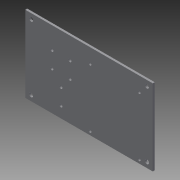
# Autodesk Inventor part: base_ps_rpi
Saved by Autodesk Inventor 2014 (Build 180170000, 170)
## iProperties
Created: 2015-04-20
Part Number: base_ps_rpi
Material: Generic
Document SubType Name: Modeling
Designer: Sousaadm
Density: 1 g/cm^3
Appearance: Default
Author: Sousaadm
Autodesk Inventor part; units mm, degrees
ref_plane "YZ Plane" through (0, 0, 0) normal (1, 0, 0) x (0, 1, 0)
ref_plane "XZ Plane" through (0, 0, 0) normal (0, 1, 0) x (-1, 0, 0)
ref_plane "XY Plane" through (0, 0, 0) normal (0, 0, 1) x (1, 0, 0)
sketch "Sketch1" plane through (0, 0, 0) normal (0, 1, 0) x (-1, 0, 0)
  line L0 (0, 0) -> (-127, 0)
  line L1 (-127, 0) -> (-127, 76)
  line L2 (-127, 76) -> (0, 76)
  line L3 (0, 76) -> (0, 0)
  dimension "d0" = 76
  dimension "d1" = 127
  constraints: 8 end point, 2 parallel, 1 horizontal, 1 perpendicular
  measures "d0" distance of L2.end L0.start
  measures "d1" distance of L1.end L2.end
extrude "Extrusion1" add sketch "Sketch1" along normal blind 2
sketch "Sketch2" plane through (0, 0, 0) normal (0, -1, 0) x (1, 0, 0)
  line L0 (0, 0) -> (127, 0) projected
  line L1 (127, 0) -> (127, 76) projected
  line L2 (127, 76) -> (0, 76) projected
  line L3 (0, 76) -> (0, 0) projected
  line L4 (0, 5.4) -> (127, 5.4) construction
  line L5 (0, 38) -> (127, 38) construction
  line L6 (63.5, 76) -> (63.5, 0) construction
  line L7 (121.2, 76) -> (121.2, 0) construction
  line L8 (0, 70.6) -> (127, 70.6) construction
  line L9 (5.8, 76) -> (5.8, 0) construction
  circle A0 centre (121.2, 70.6) radius 2
  circle A1 centre (121.2, 5.4) radius 2
  circle A2 centre (5.8, 70.6) radius 2
  circle A3 centre (5.8, 5.4) radius 2
  dimension "d5" = 32.6
  dimension "d6" = 57.7
  dimension "d7" = 4
  constraints: 12 end point, 7 symmetric about line, 6 point on line, 4 centre point, 4 midpoint, 2 perpendicular, 3 other
  measures "d5" distance between parallel lines of L4 L5
  measures "d6" distance between parallel lines of L7 L6
  measures "d7" diameter of A0
extrude "Extrusion2" cut sketch "Sketch2" against normal through all contours A0 | A1 | A2 | A3
sketch "Sketch3" plane through (0, 0, 0) normal (0, -1, 0) x (1, 0, 0)
  line L0 (0, 0) -> (127, 0) projected
  line L1 (0, 76) -> (0, 0) projected
  line L2 (10, 93) -> (61, 93)
  line L3 (61, 93) -> (61, 0)
  line L4 (61, 0) -> (10, 0)
  line L5 (10, 0) -> (10, 93)
  line L6 (61, 0) -> (117, 0)
  line L7 (117, 0) -> (117, 85)
  line L8 (117, 85) -> (61, 85)
  line L9 (61, 85) -> (61, 0)
  line L10 (35.5, 93) -> (35.5, 0) construction
  circle A0 centre (35.5, 27) radius 1.5
  circle A1 centre (35.5, 82) radius 1.5
  line L11 (89, 85) -> (89, 0) construction
  line L12 (117, 42.5) -> (61, 42.5) construction
  circle A2 centre (113.5, 3.5) radius 1.375
  circle A3 centre (113.5, 61.5) radius 1.375
  circle A4 centre (64.5, 3.5) radius 1.375
  circle A5 centre (64.5, 61.5) radius 1.375
  line L13 (35.5, 82) -> (35.5, 27) construction
  circle A6 centre (44.48, 54.5) radius 1.5
  circle A7 centre (26.52, 54.5) radius 1.5
  circle A8 centre (35.5, 11) radius 1.5
  circle A9 centre (35.5, 66) radius 1.5
  line L14 (35.5, 66) -> (35.5, 11) construction
  circle A10 centre (44.48, 38.5) radius 1.5
  circle A11 centre (26.52, 38.5) radius 1.5
  dimension "d10" = 93
  dimension "d12" = 51
  dimension "d13" = 10
  dimension "d14" = 56
  dimension "d15" = 85
  dimension "d16" = 27
  dimension "d17" = 3
  dimension "d20" = 55
  dimension "d25" = 0
  dimension "d27" = 2.75
  dimension "d31" = 58
  dimension "d34" = 49
  dimension "d39" = 3.5
  dimension "d41" = 3.5
  dimension "d42" = 3
  dimension "d43" = 8.98
  dimension "d44" = 27.5
  dimension "d45" = 3
  dimension "d46" = 55
  dimension "d47" = 3
  dimension "d48" = 27.5
  dimension "d49" = 11
  dimension "d50" = 8.98
  dimension "d51" = 8.98
  dimension "d52" = 3
  constraints: 26 end point, 12 centre point, 6 midpoint, 4 parallel, 3 collinear, 3 horizontal, 2 perpendicular, 2 point on line, 2 symmetric about line, 2 vertical, 10 other
  measures "d10" distance of L4.end L2.start
  measures "d12" distance of L2.start L2.end
  measures "d13" distance between parallel lines of L1 L5
  measures "d14" distance of L7.end L8.end
  measures "d15" distance of L6.end L7.end
  measures "d16" distance from line of L0 L13.end
  measures "d17" diameter of A0
  measures "d20" distance of L13.end L13.start
  measures "d25" distance between parallel lines of L0 L6
  measures "d27" diameter of A2
  measures "d31" distance of A2.centre A3.centre
  measures "d34" distance of A2.centre A4.centre
  measures "d39" distance from line of L6 A2.centre
  measures "d41" distance from line of L7 A2.centre
  measures "d42" diameter of A6
  measures "d43" distance from line of L10 A6.centre
  measures "d44" vertical distance of A6.centre L13.end
  measures "d45" diameter of A8
  measures "d46" distance of L14.end L14.start
  measures "d47" diameter of A10
  measures "d48" vertical distance of A10.centre L14.end
  measures "d49" distance from line of L0 L14.end
  measures "d50" distance from line of L10 A10.centre
  measures "d51" distance from line of L14 A11.centre
  measures "d52" diameter of A9
extrude "Extrusion3" cut sketch "Sketch3" against normal through all contours A0 | A1 | A2 | A3 | A4 | A5 | A6 | A7 | A8 | A10 | A11
body "Solid1"
